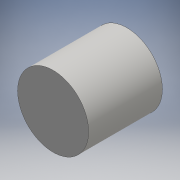
# Autodesk Inventor part: box
Saved by Autodesk Inventor 2016 (Build 200138000, 138)
## iProperties
Created: 2017-04-06
Part Number: box
Material: 一般
Document SubType Name: Modeling
Designer: Daisuke
Density: 1 g/cm^3
Appearance: 既定
Author: Daisuke
Autodesk Inventor part; units mm, degrees
ref_plane "YZ Plane" through (0, 0, 0) normal (1, 0, 0) x (0, 1, 0)
ref_plane "XZ Plane" through (0, 0, 0) normal (0, 1, 0) x (-1, 0, 0)
ref_plane "XY Plane" through (0, 0, 0) normal (0, 0, 1) x (1, 0, 0)
sketch "スケッチ1" plane through (0, 0, 0) normal (0, 1, 0) x (-1, 0, 0)
  circle A0 centre (0, 0) radius 35
  circle A1 centre (0, 0) radius 40
  dimension "d0" = 70
  dimension "d1" = 80
  constraints: 2 centre point, 2 coincident
  measures "d0" diameter of A0
  measures "d1" diameter of A1
extrude "押し出し1" add sketch "スケッチ1" along normal blind 80
sketch "スケッチ2" plane through (0, 0, 0) normal (0, -1, 0) x (1, 0, 0)
  line L0 (37.5, 1.6) -> (-37.5, 1.6)
  line L1 (-37.5, 1.6) -> (-37.5, -1.6)
  line L2 (-37.5, -1.6) -> (37.5, -1.6)
  line L3 (37.5, -1.6) -> (37.5, 1.6)
  line L4 (37.5, 1.6) -> (-37.5, -1.6) construction
  line L5 (-37.5, 1.6) -> (37.5, -1.6) construction
  line L6 (-1.6, 37.5) -> (1.6, 37.5)
  line L7 (1.6, 37.5) -> (1.6, -37.5)
  line L8 (1.6, -37.5) -> (-1.6, -37.5)
  line L9 (-1.6, -37.5) -> (-1.6, 37.5)
  line L10 (-1.6, 37.5) -> (1.6, -37.5) construction
  line L11 (1.6, 37.5) -> (-1.6, -37.5) construction
  line L12 (3.6, 38.6) -> (-3.6, 38.6)
  line L13 (-3.6, 38.6) -> (-3.6, 36.4)
  line L14 (-3.6, 36.4) -> (3.6, 36.4)
  line L15 (3.6, 36.4) -> (3.6, 38.6)
  line L16 (3.6, 38.6) -> (-3.6, 36.4) construction
  line L17 (-3.6, 38.6) -> (3.6, 36.4) construction
  line L18 (3.6, -36.4) -> (-3.6, -36.4)
  line L19 (-3.6, -36.4) -> (-3.6, -38.6)
  line L20 (-3.6, -38.6) -> (3.6, -38.6)
  line L21 (3.6, -38.6) -> (3.6, -36.4)
  line L22 (3.6, -36.4) -> (-3.6, -38.6) construction
  line L23 (-3.6, -36.4) -> (3.6, -38.6) construction
  line L24 (36.4, 3.6) -> (38.6, 3.6)
  line L25 (38.6, 3.6) -> (38.6, -3.6)
  line L26 (38.6, -3.6) -> (36.4, -3.6)
  line L27 (36.4, -3.6) -> (36.4, 3.6)
  line L28 (36.4, 3.6) -> (38.6, -3.6) construction
  line L29 (38.6, 3.6) -> (36.4, -3.6) construction
  line L30 (-36.4, 3.6) -> (-38.6, 3.6)
  line L31 (-38.6, 3.6) -> (-38.6, -3.6)
  line L32 (-38.6, -3.6) -> (-36.4, -3.6)
  line L33 (-36.4, -3.6) -> (-36.4, 3.6)
  line L34 (-36.4, 3.6) -> (-38.6, -3.6) construction
  line L35 (-38.6, 3.6) -> (-36.4, -3.6) construction
  point P0 (0, 0)
  point P1 (0, 37.5)
  point P2 (0, -37.5)
  point P3 (37.5, 0)
  point P4 (-37.5, 0)
  dimension "d4" = 75
  dimension "d5" = 3.2
  dimension "d6" = 3.2
  dimension "d7" = 75
  dimension "d8" = 7.2
  dimension "d9" = 2.2
  dimension "d10" = 7.2
  dimension "d11" = 2.2
  dimension "d12" = 2.2
  dimension "d13" = 7.2
  dimension "d14" = 2.2
  dimension "d15" = 7.2
  constraints: 72 end point, 16 midpoint, 12 parallel, 6 horizontal, 6 perpendicular
  measures "d4" distance of L2.end L1.end
  measures "d5" distance of L1.end L0.end
  measures "d6" distance of L7.end L8.end
  measures "d7" distance of L6.end L7.end
  measures "d8" distance of L14.end L13.end
  measures "d9" distance of L13.end L12.end
  measures "d10" distance of L20.end L19.end
  measures "d11" distance of L19.end L18.end
  measures "d12" distance of L25.end L26.end
  measures "d13" distance of L24.end L25.end
  measures "d14" distance of L32.end L31.end
  measures "d15" distance of L31.end L30.end
extrude "押し出し2" cut sketch "スケッチ2" against normal blind 80
sketch "スケッチ3" plane through (0, 0, 0) normal (0, -1, 0) x (1, 0, 0)
  circle A0 centre (0, 0) radius 40
  constraints: 1 centre point, 1 coincident
extrude "押し出し3" add sketch "スケッチ3" along normal blind 3
